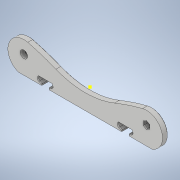
# Autodesk Inventor part: MINI-base-spoolholder
Saved by Autodesk Inventor 2021 (Build 250183000, 183)
## iProperties
Created: 2019-06-28
Material: Všeobecné
Document SubType Name: Modeling
Density: 1 g/cm^3
Appearance: Výchozí
Project: ORIGINAL PRUSA MINI
Authority: Ing. Robert Turinský
Company: Prusa Development a.s.
Author: Ing. Robert Turinský
Title: MINI-base-spoolholder
Revision Number: R4
Autodesk Inventor part; units mm, degrees
ref_plane "YZ Plane" through (0, 0, 0) normal (1, 0, 0) x (0, 1, 0)
ref_plane "XZ Plane" through (0, 0, 0) normal (0, 1, 0) x (-1, 0, 0)
ref_plane "XY Plane" through (0, 0, 0) normal (0, 0, 1) x (1, 0, 0)
sketch "Náčrt1" plane through (0, 0, 0) normal (0, 0, 1) x (1, 0, 0)
  circle A0 centre (0, 94.946) radius 100
  circle A1 centre (0, 70.5319) radius 80
  circle A2 centre (57.5, 0) radius 11
  circle A3 centre (-57.5, 0) radius 11
  line L0 (0, -257.8202) -> (0, 270.4071) projected
  line L1 (-143.9695, 0) -> (143.9695, 0) projected
  circle A4 centre (57.5, 0) radius 12
  circle A5 centre (-57.5, 0) radius 12
  line L2 (62.8852, -17) -> (-62.8852, -17)
  line L3 (-53.6594, -14.5) -> (-53.6594, -17)
  line L4 (53.6594, -14.5) -> (53.6594, -17)
  line L5 (-53.6594, -17) -> (53.6594, -17)
  circle A6 centre (0, 70.5319) radius 70
  arc A7 (-53.6594, -14.5) -> (-42.5, 0) centre (-57.5, 0) ccw
  arc A8 (42.5, 0) -> (53.6594, -14.5) centre (57.5, 0) ccw
  line L6 (-42.5, 0) -> (-39.8278, 0)
  line L7 (42.5, 0) -> (39.8278, 0)
  arc A9 (42.5, 0) -> (53.6594, -14.5) centre (57.5, 0) ccw
  arc A10 (-53.6594, -14.5) -> (-42.5, 0) centre (-57.5, 0) ccw
  arc A11 (-39.8278, 0) -> (39.8278, 0) centre (0, 70.5319) ccw
  line L8 (57.5, -3.2332) -> (54.7, -1.6166)
  line L9 (54.7, -1.6166) -> (54.7, 1.6166)
  line L10 (54.7, 1.6166) -> (57.5, 3.2332)
  line L11 (57.5, 3.2332) -> (60.3, 1.6166)
  line L12 (60.3, 1.6166) -> (60.3, -1.6166)
  line L13 (60.3, -1.6166) -> (57.5, -3.2332)
  circle A12 centre (57.5, 0) radius 3.9
  circle A13 centre (-57.5, 0) radius 3.9
  arc A14 (53.8242, 11.5426) -> (27.4981, 2.909) centre (102.8354, -182.3591) ccw
  arc A15 (-27.4981, 2.909) -> (-53.8242, 11.5426) centre (-102.8354, -182.3591) ccw
  arc A16 (-27.4981, 2.909) -> (27.4981, 2.909) centre (0, 70.5319) ccw
  line L14 (40.75, -17) -> (40.75, -15.6918)
  line L15 (40.75, -15.6918) -> (43.2521, -14.6554)
  line L16 (42.525, -11) -> (32.475, -11)
  line L17 (31.7479, -14.6554) -> (34.25, -15.6918)
  line L18 (34.25, -15.6918) -> (34.25, -17)
  line L19 (37.5, -11) -> (37.5, -6.4892)
  arc A17 (43.2521, -14.6554) -> (42.525, -11) centre (42.525, -12.9) ccw
  arc A18 (32.475, -11) -> (31.7479, -14.6554) centre (32.475, -12.9) ccw
  arc A19 (62.8852, -17) -> (53.8242, 11.5426) centre (57.5, -3) ccw
  arc A20 (-53.8242, 11.5426) -> (-62.8852, -17) centre (-57.5, -3) ccw
  circle A21 centre (57.5, 0) radius 5.25
  circle A22 centre (-57.5, 0) radius 5.25
  line L20 (44.1704, -11.95) -> (43.622, -11)
  line L21 (43.622, -11) -> (42.525, -11)
  arc A23 (44.1704, -11.95) -> (42.525, -11) centre (42.525, -12.9) ccw
  line L22 (32.475, -11) -> (31.378, -11)
  line L23 (31.378, -11) -> (30.8296, -11.95)
  arc A24 (32.475, -11) -> (30.8296, -11.95) centre (32.475, -12.9) ccw
  point P0 (0, 0)
  dimension "d0" = 200
  dimension "d1" = 160
  dimension "d2" = 22
  dimension "d3" = 115
  dimension "d10" = 24
  dimension "d11" = 17
  dimension "d13" = 10
  dimension "d18" = 1
  dimension "d35" = 5.6
  dimension "d38" = 7.8
  dimension "d45" = 200
  dimension "d46" = 7
  dimension "d47" = 135
  dimension "d48" = 13.85
  dimension "d49" = 6
  dimension "d50" = 37.5
  dimension "d51" = 1.9
  dimension "d52" = 6.5
  dimension "d63" = 3
  dimension "d64" = 15
  dimension "d65" = 2.5
  dimension "d66" = 15
  dimension "d67" = 10.5
  dimension "d114" = 60
  constraints: 44 end point, 32 point on circle, 25 centre point, 13 tangent, 10 point on line, 9 equal radius, 4 horizontal, 4 vertical, 3 coincident, 3 concentric, 3 horizontal alignment, 3 symmetric about line, 3 vertical alignment, 2 perpendicular, 1 collinear, 1 equal length, 1 midpoint, 20 other
  measures "d0" diameter of A0
  measures "d1" diameter of A1
  measures "d2" diameter of A2
  measures "d3" distance of A3.centre A2.centre
  measures "d10" diameter of A4
  measures "d11" distance from line of A2.centre L2
  measures "d13" radial gap between concentric circles of A1 A6
  measures "d18" radial gap between concentric circles of A1 A11
  measures "d35" distance between parallel lines of L9 L12
  measures "d38" diameter of A12
  measures "d45" radius of A14
  measures "d46" radial gap between concentric circles of A1 A16
  measures "d47" angle of L15 L17
  measures "d49" distance between parallel lines of L5 L16
  measures "d50" distance between parallel lines of L0 L19
  measures "d51" radius of A17
  measures "d52" distance between parallel lines of L18 L14
  measures "d63" distance from line of L1 A19.centre
  measures "d64" radius of A19
  measures "d65" distance of L4.start L4.end
  measures "d66" radius of A8
  measures "d67" diameter of A21
  measures "d114" angle of L21 L20
extrude "Vysunutí1" add sketch "Náčrt1" against normal blind 5 contours A19 A4 A0 | A0 A4 A1 A19 | A20 A1 A5 A0 | A0 A5 A20 | A4 L1 A2 A0 | A0 A1 A4 | A19 L1 A4 | A1 A4 A0 L1 A16 A14 A19 | A5 A1 A0 | A0 A3 L1 A5 | A20 A15 A16 L1 A0 A5 A1 | A5 L1 A20 | A2 A1 A0 | A2 L1 A21 | A1 A0 A4 | A4 L1 A2 | L1 A19 L2 L4 A8 A4 | A0 A1 A3 | A3 L1 A22 | A5 A0 A1 | A5 L1 A7 L3 L2 A20 | L1 A3 A5 | A1 A4 A0 | A2 L1 A21 | A2 L1 A4 A1 | A4 A1 L1 A0 | L1 A1 A4 | A0 A5 A1 | A1 A5 L1 A3 | L1 A22 A3 | A0 L1 A1 A5 | A5 A1 L1 | A21 L1 A12 | L1 A12 A21 | L1 A1 L0 A0 | A0 L0 A16 L1 | A8 L4 L2 L14 L15 A17 L20 L21 L16 L22 L23 A18 L17 L18 L0 A11 L1 | A22 L1 A13 | L1 A13 A22 | L1 A16 L0 A0 | A0 L0 A1 L1 | L1 A11 L0 L2 L3 A7 | A12 L1 L9 L8 L13 L12 | L1 L12 L11 L10 L9 A12 | L1 A11 L0 A1 | L2 L18 L17 A18 L16 A17 L15 L14 | A1 L0 A11 L1 | A13 L1 | L1 A13 | L12 L13 L8 L9 L1 | L1 L9 L10 L11 L12 | A17 L21 L20 | L23 L22 A18
extrude "Vysunutí3" add sketch "Náčrt1" against normal blind 9 contours A8 L4 L2 L14 L15 A17 L20 L21 L16 L22 L23 A18 L17 L18 L0 A11 L1 | L1 A11 L0 L2 L3 A7 | L2 L18 L17 A18 L16 A17 L15 L14 | A17 L21 L20 | L23 L22 A18
extrude "Vysunutí5" add sketch "Náčrt1" against normal blind 8.75 contours A12 L1 L9 L8 L13 L12 | L1 L12 L11 L10 L9 A12 | A13 L1 | L1 A13 | L12 L13 L8 L9 L1 | L1 L9 L10 L11 L12
extrude "Vysunutí7" add sketch "Náčrt1" against normal blind 5.5 contours A21 L1 A12 | L1 A12 A21 | A22 L1 A13 | L1 A13 A22 | A12 L1 L9 L8 L13 L12 | L1 L12 L11 L10 L9 A12 | A13 L1 | L1 A13 | L12 L13 L8 L9 L1 | L1 L9 L10 L11 L12
hole "Díra1" at (-57.5, 0, 0) direction (0, 0, -1) diameter 3.4 end through all counterbore diameter 7 counterbore depth 4.6
hole "Díra2" at (57.5, 0, 0) direction (0, 0, -1) diameter 3.4 end through all
extrude "Vysunutí4" cut sketch "Náčrt1" against normal blind 4.6 contours L12 L13 L8 L9 L1 | L1 L9 L10 L11 L12
extrude "Vysunutí6" cut sketch "Náčrt1" along normal through all both and the other way through all contours L2 L18 L17 A18 L16 A17 L15 L14 | A17 L21 L20 | L23 L22 A18
sketch "Náčrt3" plane through (0, 0, -9) normal (0, 0, -1) x (-1, 0, 0)
  line L0 (-34.25, -17) -> (53.6594, -17) projected
  line L1 (53.6594, -17) -> (53.6594, -14.5) projected
  arc A0 (42.5, 0) -> (53.6594, -14.5) centre (57.5, 0) ccw projected
  line L2 (42.5, 0) -> (39.8278, 0) projected
  arc A1 (-39.8278, 0) -> (39.8278, 0) centre (0, 70.5319) ccw projected
  line L3 (-39.8278, 0) -> (-42.5, 0) projected
  arc A2 (-53.6594, -14.5) -> (-42.5, 0) centre (-57.5, 0) ccw projected
  line L4 (-53.6594, -14.5) -> (-53.6594, -17) projected
  line L5 (-53.6594, -17) -> (-40.75, -17) projected
  line L6 (-40.75, -17) -> (-40.75, -15.6918) projected
  line L7 (-40.75, -15.6918) -> (-43.2521, -14.6554) projected
  arc A3 (-44.1704, -11.95) -> (-43.2521, -14.6554) centre (-42.525, -12.9) ccw projected
  line L8 (-43.622, -11) -> (-31.378, -11) projected
  arc A4 (-31.7479, -14.6554) -> (-30.8296, -11.95) centre (-32.475, -12.9) ccw projected
  line L9 (-31.7479, -14.6554) -> (-34.25, -15.6918) projected
  line L10 (-34.25, -15.6918) -> (-34.25, -17) projected
  line L11 (-31.378, -11) -> (-43.622, -11) projected
  line L12 (-37.5, -11) -> (-38.75, -11)
  line L13 (-40.5, 0) -> (-37.5, 0)
  line L14 (-37.5, 0) -> (-37.5, -11)
  line L15 (-39.1, -6) -> (-40.5, -6)
  line L16 (-40.5, -6) -> (-40.5, 0)
  line L17 (-38.75, -11) -> (-38.75, -7.3062)
  line L18 (-36.25, -6) -> (-34.5, -6)
  line L19 (-34.5, -6) -> (-34.5, -2.7535)
  line L20 (-36.25, -11) -> (-36.25, -6)
  line L21 (-39.1, -6) -> (-38.75, -7.3062)
  line L22 (-44.1704, -11.95) -> (-43.622, -11) projected
  line L23 (-31.378, -11) -> (-30.8296, -11.95) projected
  point P0 (0, 0)
  point P1 (-42.625, -11)
  point P2 (-32.375, -11)
  point P3 (-38.75, -6)
  dimension "d56" = 2.5
  dimension "d57" = 6
  dimension "d58" = 11
  dimension "d60" = 15
  dimension "d61" = 3.2
  constraints: 20 end point, 3 symmetric about line, 2 horizontal, 2 parallel, 2 perpendicular, 1 collinear, 1 midpoint, 1 point on circle, 3 other
  measures "d56" diameter of L17 L14
  measures "d57" diameter of L16 L14
  measures "d58" distance between parallel lines of L5 L15
  measures "d60" angle of L14 L21
  measures "d61" diameter of L15.start L14
revolve "Rotace1" cut sketch "Náčrt3" angle 360 about axis through (37.5, 0, -9) along (0, -1, 0) contours L14 L8 L17 L21 L15 L16 L3 A1 | A1 L13 L14
mirror "Zrcadlit2" about plane through (0, 0, 0) normal (1, 0, 0) of "Vysunutí6", "Rotace1"
chamfer "Zkosení3" distance 0.5 angle 60 14 edges at (40.75, -16.3459, 0) (42.001, -15.1736, 0) (44.3242, -13.5107, 0) (37.5, -11, 0) (30.6758, -13.5107, 0) (32.999, -15.1736, 0) (34.25, -16.3459, 0) (-34.25, -16.3459, 0) (-32.999, -15.1736, 0) (-30.6758, -13.5107, 0) (-37.5, -11, 0) (-44.3242, -13.5107, 0) (-42.001, -15.1736, 0) (-40.75, -16.3459, 0) measured on face at (-1.8777, -10.3693, 0)
chamfer "Zkosení5" distance 0.35 distance2 1 1 edges at (58.9, -2.4249, 0) measured on face at (-1.8777, -10.3709, 0)
chamfer "Zkosení6" distance 0.35 distance2 1 1 edges at (56.1, -2.4249, 0) measured on face at (-1.8777, -10.3709, 0)
chamfer "Zkosení7" distance 0.35 distance2 1 1 edges at (54.7, 0, 0) measured on face at (-1.8777, -10.3709, 0)
chamfer "Zkosení8" distance 0.35 distance2 1 1 edges at (56.1, 2.4249, 0) measured on face at (-1.8777, -10.3709, 0)
chamfer "Zkosení9" distance 0.35 distance2 1 1 edges at (58.9, 2.4249, 0) measured on face at (-1.8777, -10.3709, 0)
chamfer "Zkosení10" distance 0.35 distance2 1 1 edges at (60.3, 0, 0) measured on face at (-1.8777, -10.3709, 0)
fillet "Zaoblení1" [suppressed]
chamfer "Zkosení1" distance 0.3 angle 60 1 edges at (-57.5, 1.7, -4.6) measured on face at (-57.0852, -2.8496, -4.6)
chamfer "Zkosení2" distance 0.3 angle 60 1 edges at (57.5, 1.7, -4.6) measured on face at (59.9292, -0.0683, -4.6)
chamfer "Zkosení11" distance 0.5 angle 45 5 edges at (0, -2.4681, -5) (40.5115, 7.6822, -5) (71.7969, 1.5386, -5) (-40.5115, 7.6822, -5) (-71.7969, 1.5386, -5)
chamfer "Zkosení12" distance 0.25 angle 60 2 edges at (53.6, 0, -8.75) (57.5, 1.7, -8.75) measured on face at (60.6248, -0.3794, -8.75)
chamfer "Zkosení13" distance 0.25 angle 60 2 edges at (-61.4, 0, -8.75) (-57.5, 1.7, -8.75) measured on face at (-54.3752, -0.3794, -8.75)
sketch "Náčrt4" plane through (-57.5, 0, -4.6) normal (0, 0, 1) x (1, 0, 0)
  circle A0 centre (0, 0) radius 3.5 projected
  circle A1 centre (0, 0) radius 2 projected
  line L0 (115, -3.2332) -> (112.2, -1.6166) projected
  line L1 (117.8, -1.6166) -> (115, -3.2332) projected
  line L2 (117.8, 1.6166) -> (117.8, -1.6166) projected
  line L3 (115, 3.2332) -> (117.8, 1.6166) projected
  line L4 (112.2, 1.6166) -> (115, 3.2332) projected
  line L5 (112.2, -1.6166) -> (112.2, 1.6166) projected
  circle A2 centre (115, 0) radius 2 projected
  line L6 (117, 2.0785) -> (117, -2.0785)
  line L7 (113, -2.0785) -> (113, 2.0785)
  line L8 (112.8641, 2) -> (117.1359, 2)
  line L9 (117.1359, -2) -> (112.8641, -2)
  line L10 (117, 2.0785) -> (117.8, 1.6166)
  line L11 (117.8, -1.6166) -> (117, -2.0785)
  line L12 (113, -2.0785) -> (112.2, -1.6166)
  line L13 (113, 2.0785) -> (112.2, 1.6166)
  line L14 (112.8641, 2) -> (115, 3.2332)
  line L15 (115, 3.2332) -> (117.1359, 2)
  line L16 (117.1359, -2) -> (115, -3.2332)
  line L17 (115, -3.2332) -> (112.8641, -2)
  line L18 (-2.8723, 2) -> (2.8723, 2)
  line L19 (2, 2.8723) -> (2, -2.8723)
  line L20 (2.8723, -2) -> (-2.8723, -2)
  line L21 (-2, -2.8723) -> (-2, 2.8723)
  arc A3 (2.8723, 2) -> (-2.8723, 2) centre (0, 0) ccw
  arc A4 (2, -2.8723) -> (2, 2.8723) centre (0, 0) ccw
  arc A5 (-2.8723, -2) -> (2.8723, -2) centre (0, 0) ccw
  arc A6 (-2, 2.8723) -> (-2, -2.8723) centre (0, 0) ccw
  point P0 (57.5, 0)
  constraints: 32 end point, 12 point on circle, 8 point on line, 8 tangent, 4 centre point, 4 horizontal, 4 parallel, 3 vertical, 2 collinear, 1 perpendicular, 9 other
extrude "Vysunutí8" add sketch "Náčrt4" along normal blind 0.3 contours A0 L20 L19 L18 | L18 L19 A0 | A0 L19 L20 | L21 L18 A0 | A0 L20 L21 | L18 L21 L20 A0 | L0 L9 L7 | L6 L9 L1 | L0 L5 L4 L8 L7 L9 | L9 L6 L8 L3 L2 L1 | L8 L4 L7 | L6 L3 L8
extrude "Vysunutí9" add sketch "Náčrt4" along normal blind 0.6 contours L18 L19 A0 | A0 L19 L20 | L19 L18 L21 A0 | A0 L21 L20 L19 | L21 L18 A0 | A0 L20 L21 | L0 L7 L9 L6 L1 | L0 L9 L7 | L6 L9 L1 | L8 L7 L4 L3 L6 | L8 L4 L7 | L6 L3 L8
